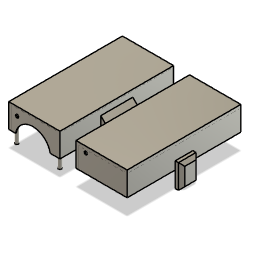
PROJECT 3D v2 (Autodesk Fusion 360 design; units mm, degrees)
Autodesk Fusion 360 part; units mm, degrees
note: some values were not read from the file. Chosen so that the rebuilt part matches the saved one: a direction; where a step starts. Set by a fixed rule: which sketch regions a step uses.
sketch "Sketch1" plane through (0, 0, 0) normal (0, 1, 0) x (1, 0, 0)
  line L0 (0, 0) -> (32, 0)
  line L1 (32, 0) -> (32, -71)
  line L2 (32, -71) -> (0, -71)
  line L3 (0, -71) -> (0, 0)
  dimension "d1" = 71
  dimension "d2" = 32
  constraint horizontal L0
  constraint vertical L1
  constraint horizontal L2
  constraint vertical L3
  constraint coincident L0.start L3.end
  measures "d1" distance of L0.start L2.end
  measures "d2" distance of L0.start L0.end
extrude "Extrude8" add sketch "Sketch1" along normal blind 30 makes body 1
ref_plane "WorkPlane5" through (16, 15, 35.5) normal (0, 1, 0) x (0, 0, 1)
split "Split1" by plane through (16, 15, 35.5) normal (0, 1, 0) bodies 1 makes body 2 at (10.6667, 30, 23.6667)
sketch "Sketch8" plane through (0, 0, 71) normal (0, 0, 1) x (1, 0, 0)
  line L0 (32, 15) -> (0, 15)
  line L1 (0, 15) -> (0, 0)
  line L2 (0, 0) -> (32, 0)
  line L3 (32, 0) -> (32, 15)
  line L4 (32, 15) -> (42, 15)
  circle A0 centre (37, 15) radius 2.5
  circle A1 centre (37, 15) radius 2.8
  circle A2 centre (37, 15) radius 4
  line L5 (32, 4.3431) -> (39.8284, 12.1716)
  line L6 (32, 25.6569) -> (39.8284, 17.8284)
  line L7 (32, 15) -> (32, 30)
  dimension "d36" = 5
  dimension "d37" = 0.3
  dimension "d38" = 8
  dimension "d39" = 5
  dimension "d40" = 45
  dimension "d41" = 45
  constraint coincident L0.start L3.end
  constraint perpendicular L3 L4
  constraint midpoint L4 A0.centre
  constraint concentric A0 A2
  constraint coincident L3 L5.start
  constraint coincident A2 L5.end
  constraint tangent A2 L5
  constraint coincident A2 L6.end
  constraint tangent A2 L6
  constraint coincident L6.start L7
  measures "d36" diameter of A0
  measures "d38" diameter of A2
  measures "d39" distance of L0.start A0.centre
  measures "d40" angle of L6 L7
  measures "d41" angle of L3 L5
extrude "Extrude10" add sketch "Sketch8" against normal blind 15 from surface at -10 contours L3 L4 A2 L5 | L4 A1 A2 | L4 A1 A2 | L4 A0 A1 | L4 A0 A1 | L4 A0 | L4 A0 bodies 1
extrude "Extrude11" add sketch "Sketch8" along normal blind 15 from surface at -61 contours L3 L4 A2 L5 | L4 A1 A2 | L4 A1 A2 | L4 A0 A1 | L4 A0 A1 | L4 A0 | L4 A0 bodies 1
extrude "Extrude12" add sketch "Sketch8" against normal blind 51 from surface at -10 contours L4 A0 | L4 A0 bodies 1
extrude "Extrude13" add sketch "Sketch8" against normal blind 20 from surface at -25.5 contours L4 A2 L6 L7 | L4 A1 A2 | L4 A1 A2 bodies 2
copy_body "Body->Comp1" bodies 2 removing the originals makes body 3 in component "Component"
copy_body "Body->Comp2" bodies 1 removing the originals makes body 4 in component "Component'"
sketch "Sketch9" plane through (2, 15, 0) normal (0, -1, 0) x (1, 0, 0)
  line L0 (72, 0) -> (72, 71)
  line L1 (72, 71) -> (40, 71)
  line L2 (40, 71) -> (40, 61)
  line L3 (40, 61) -> (39, 61)
  line L4 (39, 61) -> (39, 46)
  line L5 (39, 46) -> (40, 46)
  line L6 (40, 46) -> (40, 25)
  line L7 (40, 25) -> (39, 25)
  line L8 (39, 25) -> (39, 10)
  line L9 (39, 10) -> (40, 10)
  line L10 (40, 10) -> (40, 0)
  line L11 (40, 0) -> (72, 0)
  line L12 (71.5, 0.5) -> (41.6064, 0.5)
  line L13 (41.6064, 0.5) -> (41.6064, 70.5)
  line L14 (41.6064, 70.5) -> (71.5, 70.5)
  line L15 (71.5, 70.5) -> (71.5, 0.5)
  circle A0 centre (69, 3) radius 1
  circle A1 centre (44, 3) radius 1
  circle A2 centre (69, 68) radius 1
  circle A3 centre (44, 68) radius 1
  dimension "d58" = 70
  dimension "d59" = 29.8936
  constraint horizontal L12
  constraint vertical L13
  constraint horizontal L14
  constraint vertical L15
  measures "d58" distance of L12.end L13.end
  measures "d59" distance of L12.start L12.end
extrude "Extrude1" cut sketch "Sketch9" against normal blind 13 contours L12 L13 L14 L15 sketch seen with x (-1, 0, 0) y (0, -1, 0) z (0, 0, 1) at (74, 30, 0) bodies 4 in component "Component'"
extrude "Extrude2" cut 4 faces at (28.3434, 15, 3.2193) (3.3434, 15, 3.2193) (3.3745, 15, 68.1952) (28.3745, 15, 68.1952) along direction (0, -1, 0) blind 11 on bodies 4 bodies 4 in component "Component'"
sketch "Sketch10" plane through (0, 15, 0) normal (0, 1, 0) x (1, 0, 0)
  line L0 (1.5229, -0.5013) -> (1.5229, -70.5013)
  circle A0 centre (30, -3) radius 1
  circle A1 centre (3, -3) radius 1
  circle A2 centre (30, -69) radius 1
  circle A3 centre (3, -69) radius 1
  line L1 (31.5, -0.5) -> (1.5229, -0.5)
  line L2 (1.5229, -0.5) -> (1.5229, -70.5013)
  line L3 (1.5229, -70.5013) -> (31.5, -70.5013)
  line L4 (31.5, -70.5013) -> (31.5, -0.5)
  dimension "d64" = 70
  constraint vertical L0
  constraint horizontal L1
  constraint vertical L2
  constraint horizontal L3
  constraint vertical L4
  constraint coincident L0 L2.end
  measures "d64" distance of L0.start L0.end
extrude "Extrude1'" cut sketch "Sketch10" along normal blind 14 bodies 3 in component "Component"
extrude "Extrude2'" add 4 faces at (29.6255, 15, 2.8048) (2.6255, 15, 2.8048) (29.481, 15, 68.8122) (2.481, 15, 68.8122) along direction (0, -1, 0) blind 7 on bodies 3 bodies 3 in component "Component"
sketch "Sketch11" plane through (74, 0, 0) normal (1, 0, 0) x (0, 0, -1)
  line L0 (-71, 15) -> (0, 15)
  line L1 (0, 15) -> (0, 30)
  line L2 (0, 30) -> (-71, 30)
  line L3 (-71, 30) -> (-71, 15)
  line L4 (-30, 20) -> (-41, 20)
  line L5 (-41, 20) -> (-41, 5)
  line L6 (-41, 5) -> (-30, 5)
  line L7 (-30, 5) -> (-30, 20)
  constraint horizontal L4
  constraint vertical L5
  constraint horizontal L6
  constraint vertical L7
extrude "Extrude3" add sketch "Sketch11" along normal blind 4 contours L0 L4 L5 L7 | L0 L5 L6 L7 sketch seen with x (-1, 0, 0) y (0, -1, 0) z (0, 0, 1) at (74, 30, 0) bodies 4 in component "Component'"
chamfer "Chamfer1" distance 2 angle 45 4 edges at (-4, 25, 35.5) (-4, 17.5, 41) (-4, 17.5, 30) (-4, 10, 35.5) on bodies 4 in component "Component'"
sketch "Sketch12" plane through (74, 0, 0) normal (-1, 0, 0) x (0, 0, 1)
  line L0 (41, 15) -> (30, 15)
  line L1 (30, 15) -> (30, 5)
  line L2 (30, 5) -> (41, 5)
  line L3 (41, 5) -> (41, 15)
  line L4 (38, 5) -> (33, 5)
  line L5 (33, 5) -> (33, 7)
  line L6 (33, 7) -> (38, 7)
  line L7 (38, 7) -> (38, 5)
  dimension "d73" = 5
  dimension "d74" = 2
  constraint horizontal L4
  constraint vertical L5
  constraint horizontal L6
  constraint vertical L7
  constraint midpoint L2 L4
  measures "d73" distance of L5.end L6.end
  measures "d74" distance of L4.end L5.end
extrude "Extrude4" add sketch "Sketch12" along normal blind 1.5 contours L2 L4 L5 L6 L7 sketch seen with x (-1, 0, 0) y (0, -1, 0) z (0, 0, 1) at (74, 30, 0) bodies 4 in component "Component'"
chamfer "Chamfer2" distance 1 angle 45 4 edges at (1.5, 23, 35.5) (1.5, 24, 33) (1.5, 25, 35.5) (1.5, 24, 38) on bodies 4 in component "Component'"
sketch "Sketch13" plane through (0, 0, 0) normal (-1, 0, 0) x (0, 0, 1)
  line L0 (0, 15) -> (71, 15)
  line L1 (71, 15) -> (71, 30)
  line L2 (71, 30) -> (0, 30)
  line L3 (0, 30) -> (0, 15)
  line L4 (38.005, 22.9496) -> (33.005, 22.9496)
  line L5 (33.005, 22.9496) -> (33.005, 24.9496)
  line L6 (33.005, 24.9496) -> (38.005, 24.9496)
  line L7 (38.005, 24.9496) -> (38.005, 22.9496)
  dimension "d78" = 2
  dimension "d79" = 5
  constraint horizontal L4
  constraint vertical L5
  constraint horizontal L6
  constraint vertical L7
  measures "d78" distance of L4.start L6.end
  measures "d79" distance of L5.end L6.end
extrude "Extrude3'" cut sketch "Sketch13" against normal blind 2 contours L4 L5 L6 L7 bodies 3 in component "Component"
hole "Hole1" at (15.0773, 13.0445, 71) direction (0, 0, -1) diameter 22 depth 12 tip angle 118 bodies 3 in component "Component"
hole "Hole2" at (5.2707, 24.7681, 71) direction (0, 0, -1) diameter 2 depth 12 tip angle 118 bodies 3 in component "Component"
hole "Hole2'" at (25.8805, 3.6963, 71) direction (0, 0, -1) diameter 2 depth 12 tip angle 118 bodies 4 in component "Component'"
sketch "Sketch14" plane through (74, 30, 0) normal (0, 0, -1) x (1, 0, 0)
  line L0 (0, 15) -> (-32, 15)
  line L1 (-32, 15) -> (-32, 0)
  line L2 (-32, 0) -> (0, 0)
  line L3 (0, 0) -> (0, 15)
  line L4 (-19, 5) -> (-10.5, 5)
  line L5 (-10.5, 5) -> (-10.5, 6.5)
  line L6 (-10.5, 6.5) -> (-19, 6.5)
  line L7 (-19, 6.5) -> (-19, 5)
  constraint horizontal L4
  constraint vertical L5
  constraint horizontal L6
  constraint vertical L7
extrude "Extrude5" cut sketch "Sketch14" against normal blind 2 contours L4 L5 L6 L7 sketch seen with x (-1, 0, 0) y (0, -1, 0) z (0, 0, 1) at (74, 30, 0) bodies 4 in component "Component'"
component "Component" placed x (1, 0, 0) y (0, 1, 0) z (0, 0, 1) at (0, 0, 0)
component "Component'" placed x (-1, 0, 0) y (0, -1, 0) z (0, 0, 1) at (74, 30, 0)
